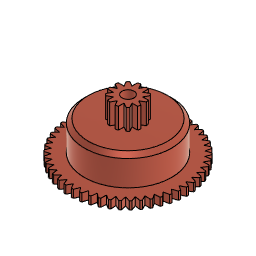
MG996R_Gear_2 v4 (Autodesk Fusion 360 design; units mm, degrees)
Autodesk Fusion 360 part; units mm, degrees
sketch "Sketch1" plane through (0, 0, 0) normal (0, 0, 1) x (1, 0, 0)
  circle A0 centre (0, 0) radius 7.5
  circle A1 centre (0, 0) radius 5.5
  circle A2 centre (0, 0) radius 2
  dimension "d1" = 15
  dimension "d2" = 11
  dimension "d3" = 4
  constraint coincident A0.centre A1.centre
  measures "d1" diameter of A0
  measures "d2" diameter of A1
  measures "d3" diameter of A2
extrude "Extrude1" add sketch "Sketch1" along normal blind 7.3 contours A2 makes body 1
extrude "Extrude2" add sketch "Sketch1" along normal blind 1 separate body contours A0 makes body 2
extrude "Extrude3" add sketch "Sketch1" along normal blind 4.7 contours A1 bodies 1 2
sketch "Sketch2" plane through (0, 0, 0) normal (0, 0, -1) x (1, 0, 0)
  circle A0 centre (0, 0) radius 7.5
  circle A1 centre (0, 0) radius 4.25
  dimension "d10" = 8.5
  constraint concentric A0 A1
  measures "d10" diameter of A1
extrude "Extrude4" cut sketch "Sketch2" against normal blind 3.5 contours A1 bodies 1
sketch "Sketch3" plane through (0, 0, 7.3) normal (0, 0, 1) x (-1, 0, 0)
  circle A0 centre (0, 0) radius 2
  circle A1 centre (0, 0) radius 0.75
  dimension "d13" = 1.5
  constraint concentric A0 A1
  measures "d13" diameter of A1
extrude "Extrude5" cut sketch "Sketch3" against normal blind 24 contours A1 bodies 1
chamfer "Chamfer1" distance 0.5 angle 45 1 edges at (-5.1278, -1.9889, 4.7) on bodies 1
sketch "Sketch4" plane through (0, 0, 7.3) normal (0, 0, 1) x (-1, 0, 0)
  circle A0 centre (0, 0) radius 0.75
  circle A1 centre (0, 0) radius 2
  circle A2 centre (0, 0) radius 2
  line L0 (0.35, -1.9691) -> (0, -1.3629)
  line L1 (0, -1.3629) -> (-0.35, -1.9691)
  dimension "d17" = 0.7
  dimension "d18" = 0.7
  constraint concentric A0 A2
  constraint coincident A2 L0.start
  constraint coincident A2 L1.end
  constraint equal L0 L1
  constraint vertical A0.centre L0.end
  constraint equal A1 A2
  measures "d17" distance of L0.start L0.end
  measures "d18" horizontal distance of L0.start L1.end
extrude "Extrude6" cut sketch "Sketch4" against normal blind 2.6 contours A1 A2 L0 L1 picked at (0, -1.7853) bodies 1
pattern_circular "C-Pattern1" count 12 over 360 about axis through (0, 0, 7.3) along (0, 0, -1) of "Extrude6"
sketch "Sketch5" plane through (0, 0, 1) normal (0, 0, 1) x (-1, 0, 0)
  circle A0 centre (0, 0) radius 5.5
  circle A1 centre (0, 0) radius 7.5
  circle A2 centre (0, 0) radius 7.5
  line L0 (0.35, -7.4918) -> (0, -6.8856)
  line L1 (0, -6.8856) -> (-0.35, -7.4918)
  dimension "d25" = 0.7
  dimension "d26" = 0.7
  constraint coincident A0.centre A1.centre
  constraint equal A1 A2
  constraint coincident A2 L0.start
  constraint coincident A2 L1.end
  constraint equal L0 L1
  constraint vertical A0.centre L0.end
  measures "d25" horizontal distance of L0.start L1.end
  measures "d26" distance of L0.start L0.end
extrude "Extrude7" cut sketch "Sketch5" against normal blind 3.5 contours A1 A2 L0 L1 picked at (0, -7.2946) bodies 1
pattern_circular "C-Pattern2" count 50 over 360 about axis through (0, 0, 7.3) along (0, 0, -1) of "Extrude7"
chamfer "Chamfer2" distance 0.5 angle 45 2 edges at (-3.9624, -1.5369, 3.5) (-3.9624, -1.5369, 0) on bodies 1
